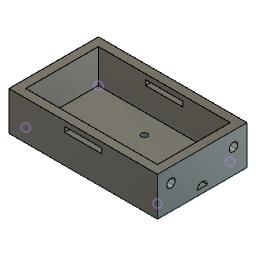
BatteryPackHolder (Autodesk Fusion 360 design; units mm, degrees)
Autodesk Fusion 360 part; units mm, degrees
sketch "Sketch1" plane through (0, 0, 0) normal (0, 1, 0) x (1, 0, 0)
  line L0 (0, 0) -> (78, 0)
  line L1 (0, 0) -> (0, -43)
  line L2 (0, -43) -> (78, -43)
  line L3 (78, 0) -> (78, -43)
  line L4 (0, 5) -> (83, 5)
  line L5 (83, 5) -> (83, -48)
  line L6 (83, -48) -> (-5, -48)
  line L7 (-5, -48) -> (-5, 5)
  line L8 (-5, 5) -> (0, 5)
  dimension "d1" = 78
  dimension "d2" = 43
  dimension "d3" = 78
  dimension "d4" = 5
  dimension "d5" = 83
  dimension "d6" = 53
  dimension "d7" = 88
  constraint coincident L0.start L1.start
  constraint horizontal L0
  constraint perpendicular L0 L1
  constraint perpendicular L1 L2
  constraint perpendicular L4 L5
  constraint perpendicular L5 L6
  constraint perpendicular L6 L7
  measures "d1" distance of L0.start L0.end
  measures "d2" distance of L0.start L1.end
  measures "d3" distance of L1.end L2.end
  measures "d4" distance of L0.start L4.start
  measures "d5" distance of L4.start L4.end
  measures "d6" distance of L4.end L5.end
  measures "d7" distance of L5.end L6.end
extrude "Extrude1" add sketch "Sketch1" along normal blind 23
sketch "Sketch2" plane through (0, 0, 0) normal (0, 1, 0) x (1, 0, 0)
sketch "Sketch3" plane through (0, 0, 0) normal (0, 1, 0) x (1, 0, 0)
  line L0 (0, 0) -> (78, 0)
  line L1 (78, 0) -> (78, -43)
  line L2 (78, -43) -> (0, -43)
  line L3 (0, -43) -> (0, 0)
  constraint horizontal L0
  constraint vertical L1
  constraint horizontal L2
  constraint vertical L3
  constraint coincident L0.start L3.end
extrude "Extrude2" add sketch "Sketch3" along normal blind 3
sketch "Sketch4" plane through (0, 3, 0) normal (0, 1, 0) x (-1, 0, 0)
  line L0 (0, 43) -> (-78, 43)
  line L1 (-78, 43) -> (-78, 0)
  line L2 (-78, 0) -> (0, 0)
sketch "Sketch5" plane through (0, 0, 0) normal (0, -1, 0) x (1, 0, 0)
  line L0 (-5, 48) -> (-5, -5)
  line L1 (-5, -5) -> (83, -5)
  line L2 (83, -5) -> (83, 48)
  line L3 (83, 48) -> (-5, 48)
sketch "Sketch6" plane through (0, 3, 0) normal (0, 1, 0) x (-1, 0, 0)
  line L0 (-39, 21.5) -> (-39, 11.75)
  line L1 (-39, 21.5) -> (-39, 31.25)
  circle A0 centre (-39, 11.75) radius 1.75
  circle A1 centre (-39, 31.25) radius 1.75
  dimension "d12" = 9.75
  dimension "d13" = 9.75
  dimension "d14" = 3.5
  dimension "d15" = 3.5
  constraint vertical L0
  constraint parallel L0 L1
  constraint coincident L0.end A0.centre
  constraint coincident L1.end A1.centre
  measures "d12" distance of L0.start L0.end
  measures "d13" distance of L0.start L1.end
  measures "d14" diameter of A0
  measures "d15" diameter of A1
extrude "Extrude3" cut sketch "Sketch6" against normal blind 20
sketch "Sketch7" plane through (0, 3, 0) normal (0, 1, 0) x (-1, 0, 0)
  circle A0 centre (-39, 11.75) radius 1.75
  circle A1 centre (-39, 31.25) radius 1.75
  line L0 (0, 43) -> (-78, 43)
  line L1 (-78, 0) -> (0, 0)
  line L2 (0, 0) -> (0, 43)
sketch "Sketch8" plane through (0, 3, 0) normal (0, 1, 0) x (-1, 0, 0)
sketch "Sketch9" plane through (83, 0, 0) normal (1, 0, 0) x (0, 0, -1)
  line L0 (-48, 0) -> (5, 0)
  line L1 (5, 0) -> (5, 23)
  line L2 (5, 23) -> (-48, 23)
  line L3 (-48, 23) -> (-48, 0)
sketch "Sketch10" plane through (83, 0, 0) normal (1, 0, 0) x (0, 0, -1)
  line L0 (-48, 0) -> (-48, 3)
  line L1 (5, 3) -> (-21.5, 3)
  line L2 (-21.5, 3) -> (-24.5, 3)
  arc A0 (-18.5, 3) -> (-24.5, 3) centre (-21.5, 3) ccw
  dimension "d18" = 3
  dimension "d19" = 6
  constraint vertical L0
  constraint coincident L1.end L2.start
  constraint parallel L1 L2
  constraint coincident L1 A0.start
  measures "d18" distance of L0.start L0.end
  measures "d19" diameter of A0
extrude "Extrude4" cut sketch "Sketch10" against normal blind 20
sketch "Sketch11" plane through (83, 0, 0) normal (1, 0, 0) x (0, 0, -1)
  line L0 (-21.5, 3) -> (-21.5, 6)
  line L1 (-21.5, 6) -> (-21.5, 23)
  line L2 (-21.5, 23) -> (-21.5, 14.5)
  circle A0 centre (-40, 14.5) radius 2.5
  line L3 (-21.5, 14.5) -> (-3, 14.5)
  circle A1 centre (-3, 14.5) radius 2.5
  dimension "d22" = 5
  dimension "d24" = 18.5
  dimension "d25" = 5
  constraint vertical L0
  constraint parallel L0 L1
  constraint midpoint L1 L2.end
  constraint perpendicular L2 L3
  constraint coincident L3.end A1.centre
  measures "d22" diameter of A0
  measures "d24" distance of L2.end L3.end
  measures "d25" diameter of A1
extrude "Extrude5" cut sketch "Sketch11" against normal blind 50
sketch "Sketch12" plane through (0, 0, -5) normal (0, 0, -1) x (-1, 0, 0)
  line L0 (-83, 0) -> (5, 0)
  line L1 (5, 0) -> (5, 23)
  line L2 (5, 23) -> (-83, 23)
  line L3 (-83, 23) -> (-83, 0)
  line L4 (-39, 20) -> (-50, 20)
  line L5 (-50, 20) -> (-50, 17)
  line L6 (-50, 17) -> (-28, 17)
  line L7 (-28, 17) -> (-28, 20)
  line L8 (-28, 20) -> (-39, 20)
  dimension "d29" = 3
  dimension "d30" = 22
  constraint perpendicular L5 L6
  constraint perpendicular L6 L7
  constraint perpendicular L7 L8
  measures "d29" distance of L4.end L5.end
  measures "d30" distance of L5.end L6.end
extrude "Extrude6" cut sketch "Sketch12" against normal blind 100 contours L4 L5 L6 L7 L8
